Autodesk Fusion 360 part; units mm, degrees
note: some values were not read from the file. Chosen so that the rebuilt part matches the saved one: a direction. Set by a fixed rule: which sketch regions a step uses.
(part 8 of 8)
  spline S20 degree 5 poles (-55.9921, 8.7646) (-55.9937, 8.7687) (-55.9971, 8.7768) (-56.0026, 8.7889) (-56.0105, 8.8046) (-56.0215, 8.8237) (-56.0332, 8.8426) (-56.0453, 8.8612) (-56.0577, 8.8797) (-56.0702, 8.8982) (-56.0829, 8.9166) (-56.0959, 8.9349) (-56.1091, 8.953) (-56.1227, 8.971) (-56.1367, 8.9888) (-56.1509, 9.0065) (-56.1655, 9.024) (-56.1802, 9.0413) (-56.1952, 9.0586) (-56.2104, 9.0758) (-56.2258, 9.0929) (-56.2413, 9.1098) (-56.2571, 9.1267) (-56.2731, 9.1434) (-56.2893, 9.16) (-56.3058, 9.1765) (-56.3224, 9.1929) (-56.3392, 9.2092) (-56.3562, 9.2254) (-56.3734, 9.2414) (-56.3907, 9.2574) (-56.4082, 9.2732) (-56.4259, 9.289) (-56.4438, 9.3046) (-56.4618, 9.3202) (-56.48, 9.3356) (-56.4984, 9.3509) (-56.5169, 9.3661) (-56.5356, 9.3813) (-56.5544, 9.3963) (-56.5735, 9.4112) (-56.5926, 9.426) (-56.6119, 9.4407) (-56.6314, 9.4552) (-56.651, 9.4697) (-56.6707, 9.4841) (-56.6906, 9.4984) (-56.7107, 9.5126) (-56.7309, 9.5266) (-56.7512, 9.5406) (-56.7717, 9.5545) (-56.7923, 9.5682) (-56.813, 9.5819) (-56.8339, 9.5954) (-56.8549, 9.6088) (-56.8761, 9.6222) (-56.8974, 9.6354) (-56.9188, 9.6485) (-56.9403, 9.6615) (-56.962, 9.6744) (-56.9838, 9.6872) (-57.0057, 9.6999) (-57.0278, 9.7125) (-57.05, 9.725) (-57.0723, 9.7374) (-57.0947, 9.7497) (-57.1172, 9.7618) (-57.1399, 9.7739) (-57.1626, 9.7858) (-57.1855, 9.7977) (-57.2086, 9.8094) (-57.2271, 9.8187) (-57.241, 9.8256) (-57.2503, 9.8302) (-57.255, 9.8325) knots 0 0 0 0 0 0 0.01428571 0.02857143 0.04285714 0.05714286 0.07142857 0.08571429 0.1 0.11428571 0.12857143 0.14285714 0.15714286 0.17142857 0.18571429 0.2 0.21428571 0.22857143 0.24285714 0.25714286 0.27142857 0.28571429 0.3 0.31428571 0.32857143 0.34285714 0.35714286 0.37142857 0.38571429 0.4 0.41428571 0.42857143 0.44285714 0.45714286 0.47142857 0.48571429 0.5 0.51428571 0.52857143 0.54285714 0.55714286 0.57142857 0.58571429 0.6 0.61428571 0.62857143 0.64285714 0.65714286 0.67142857 0.68571429 0.7 0.71428571 0.72857143 0.74285714 0.75714286 0.77142857 0.78571429 0.8 0.81428571 0.82857143 0.84285714 0.85714286 0.87142857 0.88571429 0.9 0.91428571 0.92857143 0.94285714 0.95714286 0.97142857 0.98571429 1 1 1 1 1 1
  arc A42 (-57.255, 9.8325) -> (-57.8462, 9.4911) centre (-53.7044, 3) ccw
  spline S21 degree 5 poles (-57.8462, 9.4911) (-57.8466, 9.486) (-57.8473, 9.4756) (-57.8482, 9.4601) (-57.8494, 9.4394) (-57.8508, 9.4136) (-57.852, 9.3879) (-57.853, 9.3622) (-57.8539, 9.3365) (-57.8546, 9.3109) (-57.8552, 9.2854) (-57.8556, 9.2599) (-57.8559, 9.2344) (-57.856, 9.209) (-57.856, 9.1837) (-57.8558, 9.1584) (-57.8555, 9.1332) (-57.855, 9.108) (-57.8543, 9.0829) (-57.8535, 9.0579) (-57.8525, 9.0329) (-57.8514, 9.008) (-57.8501, 8.9831) (-57.8487, 8.9583) (-57.8471, 8.9336) (-57.8453, 8.9089) (-57.8434, 8.8843) (-57.8413, 8.8598) (-57.839, 8.8354) (-57.8366, 8.811) (-57.834, 8.7867) (-57.8313, 8.7625) (-57.8284, 8.7383) (-57.8253, 8.7143) (-57.8221, 8.6903) (-57.8187, 8.6664) (-57.8151, 8.6425) (-57.8114, 8.6188) (-57.8075, 8.5951) (-57.8034, 8.5716) (-57.7991, 8.5481) (-57.7947, 8.5247) (-57.7901, 8.5014) (-57.7853, 8.4782) (-57.7803, 8.4551) (-57.7751, 8.4321) (-57.7698, 8.4092) (-57.7643, 8.3864) (-57.7586, 8.3637) (-57.7527, 8.3411) (-57.7467, 8.3187) (-57.7404, 8.2963) (-57.7339, 8.2741) (-57.7272, 8.252) (-57.7203, 8.23) (-57.7132, 8.2082) (-57.7059, 8.1864) (-57.6984, 8.1648) (-57.6908, 8.1433) (-57.6829, 8.122) (-57.6747, 8.1008) (-57.6663, 8.0798) (-57.6575, 8.0591) (-57.6484, 8.0385) (-57.639, 8.0182) (-57.6295, 7.998) (-57.6197, 7.9779) (-57.6099, 7.9579) (-57.5998, 7.9381) (-57.5893, 7.9185) (-57.5782, 7.8995) (-57.5686, 7.8847) (-57.5609, 7.874) (-57.5556, 7.867) (-57.5528, 7.8635) knots -1 -1 -1 -1 -1 -1 -0.98571429 -0.97142857 -0.95714286 -0.94285714 -0.92857143 -0.91428571 -0.9 -0.88571429 -0.87142857 -0.85714286 -0.84285714 -0.82857143 -0.81428571 -0.8 -0.78571429 -0.77142857 -0.75714286 -0.74285714 -0.72857143 -0.71428571 -0.7 -0.68571429 -0.67142857 -0.65714286 -0.64285714 -0.62857143 -0.61428571 -0.6 -0.58571429 -0.57142857 -0.55714286 -0.54285714 -0.52857143 -0.51428571 -0.5 -0.48571429 -0.47142857 -0.45714286 -0.44285714 -0.42857143 -0.41428571 -0.4 -0.38571429 -0.37142857 -0.35714286 -0.34285714 -0.32857143 -0.31428571 -0.3 -0.28571429 -0.27142857 -0.25714286 -0.24285714 -0.22857143 -0.21428571 -0.2 -0.18571429 -0.17142857 -0.15714286 -0.14285714 -0.12857143 -0.11428571 -0.1 -0.08571429 -0.07142857 -0.05714286 -0.04285714 -0.02857143 -0.01428571 0 0 0 0 0 0
  line L21 (-57.5528, 7.8635) -> (-57.0716, 7.2553)
  arc A43 (-57.0865, 7.116) -> (-57.0716, 7.2553) centre (-57.15, 7.1933) ccw
  arc A44 (-57.0865, 7.116) -> (-57.8204, 6.3821) centre (-53.7044, 3) ccw
  arc A45 (-57.9597, 6.3672) -> (-57.8204, 6.3821) centre (-57.8977, 6.4456) ccw
  line L22 (-57.9597, 6.3672) -> (-58.5679, 6.8484)
  spline S22 degree 5 poles (-58.5679, 6.8484) (-58.5714, 6.8512) (-58.5784, 6.8565) (-58.5891, 6.8642) (-58.6039, 6.8738) (-58.6229, 6.8849) (-58.6425, 6.8954) (-58.6623, 6.9055) (-58.6823, 6.9154) (-58.7023, 6.9251) (-58.7226, 6.9346) (-58.7429, 6.944) (-58.7635, 6.9531) (-58.7842, 6.9619) (-58.8052, 6.9703) (-58.8264, 6.9785) (-58.8477, 6.9864) (-58.8692, 6.994) (-58.8908, 7.0015) (-58.9126, 7.0088) (-58.9344, 7.0159) (-58.9564, 7.0228) (-58.9785, 7.0295) (-59.0007, 7.036) (-59.023, 7.0423) (-59.0455, 7.0483) (-59.0681, 7.0542) (-59.0908, 7.0599) (-59.1136, 7.0654) (-59.1365, 7.0708) (-59.1595, 7.0759) (-59.1826, 7.0809) (-59.2058, 7.0857) (-59.2291, 7.0903) (-59.2525, 7.0947) (-59.2759, 7.099) (-59.2995, 7.1031) (-59.3232, 7.107) (-59.3469, 7.1107) (-59.3707, 7.1143) (-59.3947, 7.1177) (-59.4186, 7.1209) (-59.4427, 7.124) (-59.4669, 7.1269) (-59.4911, 7.1297) (-59.5154, 7.1322) (-59.5398, 7.1346) (-59.5642, 7.1369) (-59.5887, 7.139) (-59.6133, 7.1409) (-59.638, 7.1427) (-59.6627, 7.1443) (-59.6875, 7.1457) (-59.7123, 7.147) (-59.7373, 7.1481) (-59.7622, 7.1491) (-59.7873, 7.1499) (-59.8124, 7.1506) (-59.8376, 7.1511) (-59.8628, 7.1514) (-59.8881, 7.1516) (-59.9134, 7.1516) (-59.9388, 7.1515) (-59.9642, 7.1513) (-59.9897, 7.1508) (-60.0153, 7.1502) (-60.0409, 7.1495) (-60.0665, 7.1486) (-60.0922, 7.1476) (-60.118, 7.1464) (-60.1438, 7.145) (-60.1645, 7.1438) (-60.18, 7.1429) (-60.1904, 7.1422) (-60.1955, 7.1419) knots 0 0 0 0 0 0 0.01428571 0.02857143 0.04285714 0.05714286 0.07142857 0.08571429 0.1 0.11428571 0.12857143 0.14285714 0.15714286 0.17142857 0.18571429 0.2 0.21428571 0.22857143 0.24285714 0.25714286 0.27142857 0.28571429 0.3 0.31428571 0.32857143 0.34285714 0.35714286 0.37142857 0.38571429 0.4 0.41428571 0.42857143 0.44285714 0.45714286 0.47142857 0.48571429 0.5 0.51428571 0.52857143 0.54285714 0.55714286 0.57142857 0.58571429 0.6 0.61428571 0.62857143 0.64285714 0.65714286 0.67142857 0.68571429 0.7 0.71428571 0.72857143 0.74285714 0.75714286 0.77142857 0.78571429 0.8 0.81428571 0.82857143 0.84285714 0.85714286 0.87142857 0.88571429 0.9 0.91428571 0.92857143 0.94285714 0.95714286 0.97142857 0.98571429 1 1 1 1 1 1
  arc A46 (-60.1955, 7.1419) -> (-60.5369, 6.5506) centre (-53.7044, 3) ccw
  spline S23 degree 5 poles (-60.5369, 6.5506) (-60.5346, 6.5459) (-60.53, 6.5366) (-60.5231, 6.5227) (-60.5138, 6.5042) (-60.5021, 6.4812) (-60.4902, 6.4583) (-60.4783, 6.4355) (-60.4662, 6.4128) (-60.4541, 6.3903) (-60.4418, 6.3679) (-60.4294, 6.3456) (-60.4169, 6.3234) (-60.4043, 6.3013) (-60.3916, 6.2794) (-60.3788, 6.2576) (-60.3659, 6.2359) (-60.3529, 6.2144) (-60.3398, 6.193) (-60.3266, 6.1717) (-60.3132, 6.1506) (-60.2998, 6.1295) (-60.2862, 6.1087) (-60.2726, 6.0879) (-60.2588, 6.0673) (-60.245, 6.0468) (-60.231, 6.0265) (-60.217, 6.0063) (-60.2028, 5.9863) (-60.1885, 5.9664) (-60.1741, 5.9466) (-60.1596, 5.927) (-60.145, 5.9075) (-60.1304, 5.8882) (-60.1156, 5.8691) (-60.1006, 5.8501) (-60.0856, 5.8312) (-60.0705, 5.8125) (-60.0553, 5.794) (-60.04, 5.7756) (-60.0246, 5.7574) (-60.009, 5.7394) (-59.9934, 5.7215) (-59.9776, 5.7038) (-59.9618, 5.6863) (-59.9458, 5.669) (-59.9298, 5.6518) (-59.9136, 5.6348) (-59.8973, 5.618) (-59.8809, 5.6014) (-59.8644, 5.585) (-59.8478, 5.5687) (-59.8311, 5.5527) (-59.8142, 5.537) (-59.7973, 5.5214) (-59.7802, 5.506) (-59.763, 5.4908) (-59.7457, 5.4759) (-59.7283, 5.4611) (-59.7108, 5.4465) (-59.6932, 5.4323) (-59.6754, 5.4183) (-59.6574, 5.4047) (-59.6393, 5.3915) (-59.621, 5.3785) (-59.6026, 5.3658) (-59.5841, 5.3533) (-59.5656, 5.3409) (-59.5469, 5.3288) (-59.5281, 5.3171) (-59.5089, 5.3062) (-59.4933, 5.2982) (-59.4812, 5.2927) (-59.4731, 5.2894) (-59.469, 5.2877) knots -1 -1 -1 -1 -1 -1 -0.98571429 -0.97142857 -0.95714286 -0.94285714 -0.92857143 -0.91428571 -0.9 -0.88571429 -0.87142857 -0.85714286 -0.84285714 -0.82857143 -0.81428571 -0.8 -0.78571429 -0.77142857 -0.75714286 -0.74285714 -0.72857143 -0.71428571 -0.7 -0.68571429 -0.67142857 -0.65714286 -0.64285714 -0.62857143 -0.61428571 -0.6 -0.58571429 -0.57142857 -0.55714286 -0.54285714 -0.52857143 -0.51428571 -0.5 -0.48571429 -0.47142857 -0.45714286 -0.44285714 -0.42857143 -0.41428571 -0.4 -0.38571429 -0.37142857 -0.35714286 -0.34285714 -0.32857143 -0.31428571 -0.3 -0.28571429 -0.27142857 -0.25714286 -0.24285714 -0.22857143 -0.21428571 -0.2 -0.18571429 -0.17142857 -0.15714286 -0.14285714 -0.12857143 -0.11428571 -0.1 -0.08571429 -0.07142857 -0.05714286 -0.04285714 -0.02857143 -0.01428571 0 0 0 0 0 0
  line L23 (-59.469, 5.2877) -> (-58.7481, 5.0016)
  arc A47 (-58.6914, 4.8735) -> (-58.7481, 5.0016) centre (-58.785, 4.9087) ccw
  circle A48 centre (-53.7044, 3) radius 1.5
  circle A49 centre (-53.7044, 3) radius 8.5
  dimension "d174" = 17
  constraint concentric A0 A49
  measures "d174" diameter of A49
extrude "Extrude3''" add sketch "Sketch8" along normal blind 5 contours A0 A1 L0 S0 A2 S1 L1 A3 A4 A5 L2 S2 A6 S3 L3 A7 A8 A9 L4 S4 A10 S5 L5 A11 A12 A13 L6 S6 A14 S7 L7 A15 A16 A17 L8 S8 A18 S9 L9 A19 A20 A21 L10 S10 A22 S11 L11 A23 A24 A25 L12 S12 A26 S13 L13 A27 A28 A29 L14 S14 A30 S15 L15 A31 A32 A33 L16 S16 A34 S17 L17 A35 A36 A37 L18 S18 A38 S19 L19 A39 A40 A41 L20 S20 A42 S21 L21 A43 A44 A45 L22 S22 A46 S23 L23 A47 | A49 sketch seen with x (1, 0, 0) y (0, 0, 1) z (0, -1, 0) at (-53.7044, 3, -59.3924) bodies 10 in component "Spur Gear 12 teeth"
component "Component'" placed x (-0.000786, 0, -1) y (0, 1, 0) z (1, 0, -0.000786) at (4.7617, 3, -56.0079)
component "Spur Gear 24 teeth" placed x (0, 0, -1) y (-1, 0, 0) z (0, 1, 0) at (-13.5, 3, -37.5997)
component "Component''" placed x (1, 0, 0) y (0, 1, 0) z (0, 0, 1) at (0, 0, 0)
component "Component" placed x (0.374356, 0, -0.927285) y (0, 1, 0) z (0.927285, 0, 0.374356) at (-13.5, 0, -68.5997)
component "Spur Gear 24 teeth (1)" placed x (-0.79371, 0, -0.608296) y (-0.608296, 0, 0.79371) z (0, 1, 0) at (13.5, 3, -37.5997)
component "Component1(Mirror)" placed x (-0.374353, 0, -0.927286) y (0, 1, 0) z (0.927286, 0, -0.374353) at (13.4728, 0, -68.5997)
component "Component2(Mirror)" placed x (-0.000089, 0, -1) y (0, 1, 0) z (1, 0, -0.000089) at (-4.76, 3, -55.9991)
component "Component''" placed x (1, 0, 0) y (0, 1, 0) z (0, 0, 1) at (0, -3, 0)
component "Component'" placed x (-0.000876, 0, -1) y (0, 1, 0) z (1, 0, -0.000876) at (23.5017, -6, -35.6085)
component "Component'" placed x (-0.000089, 0, -1) y (0, 1, 0) z (1, 0, -0.000089) at (15.24, -6, -56.0009)
component "Component'" placed x (-0.000786, 0, -1) y (0, 1, 0) z (1, 0, -0.000786) at (4.7617, -6, -56.0079)
component "Component'" placed x (0, 0, -1) y (0, 1, 0) z (1, 0, 0) at (-3.5, -6, -35.5997)
component "Component1(Mirror)" placed x (-0.374353, 0, -0.927286) y (0, 1, 0) z (0.927286, 0, -0.374353) at (13.4728, -3, -68.5997)
component "Component" placed x (0.374356, 0, -0.927285) y (0, 1, 0) z (0.927285, 0, 0.374356) at (-13.5, -3, -68.5997)
component "Component'''" placed x (0.79371, 0, 0.608296) y (0, 1, 0) z (-0.608296, 0, 0.79371) at (-30.1541, -28, -71.056)
component "Component'''" placed x (1, 0, -0.000089) y (0, 1, 0) z (0.000089, 0, 1) at (-49.7602, -28, -57.9951)
component "Component'''" placed x (1, 0, -0.000089) y (0, 1, 0) z (0.000089, 0, 1) at (-49.7629, -28, -88.9951)
component "Component'''" placed x (1, 0, 0) y (0, 1, 0) z (0, 0, 1) at (-68.5, -28, -37.5997)
component "Component'''" placed x (1, 0, -0.000786) y (0, 1, 0) z (0.000786, 0, 1) at (-60.2398, -28, -57.9568)
component "Component'''" placed x (0.79371, 0, 0.608296) y (0, 1, 0) z (-0.608296, 0, 0.79371) at (-30.1812, -28, -102.056)
component "Component'''" placed x (1, 0, 0) y (0, 1, 0) z (0, 0, 1) at (-68.5, -28, -68.5997)
component "Component'''" placed x (1, 0, -0.000786) y (0, 1, 0) z (0.000786, 0, 1) at (-60.2642, -28, -88.9568)
component "Spur Gear 12 teeth" placed x (0.984785, 0, -0.173777) y (0.173777, 0, 0.984785) z (0, -1, 0) at (7.5, 9, -17.5997)
